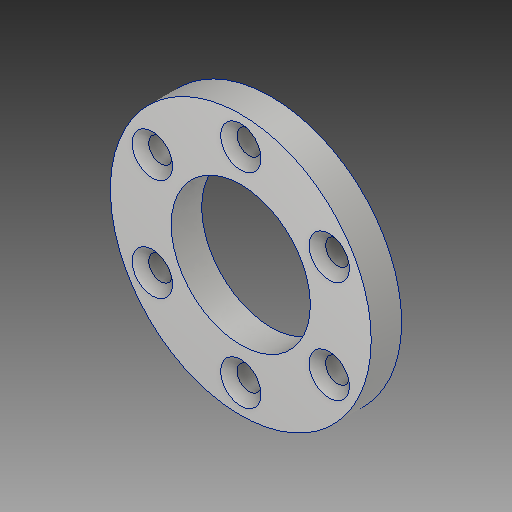
# Autodesk Inventor part: Bearing Block
Saved by Autodesk Inventor 2019.4 (Build 234330000, 330)
## iProperties
Created: 2020-01-05
Part Number: Bearing Block
Material: Aluminum 6061
Document SubType Name: Modeling
Designer: Mark
Mass: 34.9224 g
Surface Area: 64.2296 cm^2
Volume: 12.9342 cm^3
Density: 2.7 g/cm^3
Appearance: Aluminum - Flat
Author: Mark
Autodesk Inventor part; units mm, degrees
ref_plane "YZ Plane" through (0, 0, 0) normal (1, 0, 0) x (0, 1, 0)
ref_plane "XZ Plane" through (0, 0, 0) normal (0, 1, 0) x (-1, 0, 0)
ref_plane "XY Plane" through (0, 0, 0) normal (0, 0, 1) x (1, 0, 0)
sketch "Sketch1" plane through (0, 0, 0) normal (0, 0, 1) x (1, 0, 0)
  circle A0 centre (0, 0) radius 16
  circle A1 centre (0, 0) radius 30
  circle A2 centre (0, 0) radius 23.5 construction
  line L0 (0, 0) -> (0, 23.5) construction
  line L1 (0, 0) -> (23.5, 0) construction
  circle A3 centre (0, 23.5) radius 2.75
  line L2 (0, 0) -> (-20.3516, 11.75) construction
  circle A4 centre (-20.3516, 11.75) radius 2.75
  line L3 (0, 0) -> (-20.3516, -11.75) construction
  circle A5 centre (-20.3516, -11.75) radius 2.75
  line L4 (0, 0) -> (0, -23.5) construction
  circle A6 centre (0, -23.5) radius 2.75
  line L5 (0, 0) -> (20.3516, -11.75) construction
  circle A7 centre (20.3516, -11.75) radius 2.75
  line L6 (0, 0) -> (20.3516, 11.75) construction
  circle A8 centre (20.3516, 11.75) radius 2.75
  dimension "d2" = 47
  dimension "d0" = 32
  dimension "d1" = 60
  dimension "d3" = 90
  dimension "d4" = 5.5
  dimension "d7" = 360
  constraints: 14 end point, 9 coincident, 8 centre point, 1 horizontal, 1 perpendicular, 1 vertical alignment, 33 other
  measures "d0" diameter of A0
  measures "d1" diameter of A1
  measures "d3" angle of L1 L0
  measures "d4" diameter of A3
extrude "Extrusion1" add sketch "Sketch1" along normal blind 7
sketch "Sketch2" plane through (0, 0, 7) normal (0, 0, 1) x (1, 0, 0)
  circle A0 centre (-20.3516, 11.75) radius 2.75 projected
  circle A1 centre (0, 23.5) radius 2.75 projected
  circle A2 centre (20.3516, 11.75) radius 2.75 projected
  circle A3 centre (20.3516, -11.75) radius 2.75 projected
  circle A4 centre (0, -23.5) radius 2.75 projected
  circle A5 centre (-20.3516, -11.75) radius 2.75 projected
  point P0 (0, 0)
hole "Hole1" at (-20.3516, 11.75, 7) at (0, 23.5, 7) at (20.3516, 11.75, 7) at (20.3516, -11.75, 7) at (0, -23.5, 7) at (-20.3516, -11.75, 7) direction (0, 0, -1) diameter 5.5 depth 7 countersink diameter 9.3 countersink angle 90
body "Solid1"
